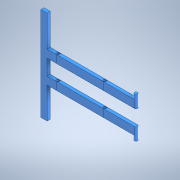
# Autodesk Inventor part: base
Saved by Autodesk Inventor 2022 (Build 260153000, 153)
## iProperties
Created: 2021-12-27
Part Number: base
Material: Stainless Steel
Document SubType Name: Modeling
Designer: G S SHOURIE
Density: 8 g/cm^3
Appearance: Cyan
Mass: 1571.73 g
Surface Area: 614.982 cm^2
Volume: 196.466 cm^3
Author: G S SHOURIE
Autodesk Inventor part; units mm, degrees
ref_plane "YZ Plane" through (0, 0, 0) normal (1, 0, 0) x (0, 1, 0)
ref_plane "XZ Plane" through (0, 0, 0) normal (0, 1, 0) x (-1, 0, 0)
ref_plane "XY Plane" through (0, 0, 0) normal (0, 0, 1) x (1, 0, 0)
sketch "Sketch1" plane through (0, 0, 0) normal (0, 0, 1) x (1, 0, 0)
  line L0 (-150, 150) -> (150, 150)
  line L1 (150, 150) -> (150, -150)
  line L2 (150, -150) -> (-150, -150)
  line L3 (-150, -150) -> (-150, 150)
  point P0 (0, 0)
  dimension "d0" = 300
  dimension "d1" = 300
  dimension "d2" = 150
  dimension "d3" = 150
  constraints: 8 end point, 2 parallel, 1 horizontal, 1 perpendicular
  measures "d0" distance of L0.start L0.end
  measures "d1" distance of L0.end L1.end
  measures "d2" distance from line of L3 point (0, 0)
  measures "d3" distance from line of L0 point (0, 0)
extrude "Extrusion1" add sketch "Sketch1" along normal mid plane 10
sketch "Sketch2" plane through (0, 0, 5) normal (0, 0, 1) x (1, 0, 0)
  line L0 (-130, 25) -> (323.6487, 25)
  line L1 (323.6487, 25) -> (323.6487, -25)
  line L2 (323.6487, -25) -> (-130, -25)
  line L3 (-130, -25) -> (-130, 25)
  point P0 (0, 0)
  dimension "d6" = 50
  dimension "d7" = 25
  dimension "d8" = 130
  constraints: 8 end point, 2 parallel, 1 horizontal, 1 perpendicular
  measures "d6" distance of L0.end L1.end
  measures "d7" distance from line of L0 point (0, 0)
  measures "d8" distance from line of L3 point (0, 0)
extrude "Extrusion2" cut sketch "Sketch2" against normal blind 10
sketch "Sketch3" plane through (0, 0, 5) normal (0, 0, 1) x (1, 0, 0)
  line L0 (170, -50) -> (-130, -50)
  line L1 (-130, -50) -> (-130, -158.2485)
  line L2 (-130, -158.2485) -> (170, -158.2485)
  line L3 (170, -158.2485) -> (170, -50)
  line L4 (150, -25) -> (-130, -25) projected
  point P0 (0, 0)
  dimension "d11" = 300
  dimension "d12" = 130
  dimension "d13" = 25
  constraints: 8 end point, 2 parallel, 1 horizontal, 1 perpendicular
  measures "d11" distance of L1.end L2.end
  measures "d12" distance from line of L1 point (0, 0)
  measures "d13" distance between parallel lines of L0 L4
extrude "Extrusion3" cut sketch "Sketch3" against normal blind 10
mirror "Mirror1" about plane through (0, 0, 0) normal (0, 1, 0) of "Extrusion3"
sketch "Sketch4" plane through (-130, -50, 5) normal (0, -1, 0) x (1, 0, 0)
  point P0 (130, -5)
sketch "Sketch5" plane through (-130, -50, 5) normal (0, -1, 0) x (1, 0, 0)
  point P0 (130, -5)
sketch "Sketch6" plane through (-130, -50, 5) normal (0, -1, 0) x (1, 0, 0)
  point P0 (130, -5)
sketch "Sketch7" plane through (-130, 25, 5) normal (0, -1, 0) x (1, 0, 0)
  circle A0 centre (30, -5) radius 5
  line L0 (0, -10) -> (280, -10) projected
  point P0 (130, -5)
  dimension "d16" = 100
  dimension "d17" = 10
  constraints: 1 centre point, 1 tangent
  measures "d16" distance of A0.centre point (130, -5)
  measures "d17" diameter of A0
extrude "Extrusion4" cut sketch "Sketch7" against normal up to surface (25 mm away)
mirror "Mirror2" about plane through (0, 0, 0) normal (0, 1, 0) of "Extrusion4"
sketch "Sketch8" plane through (-130, -50, 5) normal (0, -1, 0) x (1, 0, 0)
  line L0 (280, 0) -> (280, -10) projected
  circle A0 centre (280, -5) radius 5
  line L1 (0, 0) -> (280, 0) projected
  point P0 (130, -5)
  constraints: 1 centre point, 1 midpoint, 1 tangent
extrude "Extrusion5" add sketch "Sketch8" along normal blind 15
sketch "Sketch9" plane through (-130, -50, 5) normal (0, 1, 0) x (1, 0, 0)
  line L0 (280, 10) -> (280, 0) projected
  circle A0 centre (280, 5) radius 5
  point P0 (130, 5)
  constraints: 1 centre point, 1 midpoint
extrude "Extrusion6" add sketch "Sketch9" along normal up to surface (25 mm away)
mirror "Mirror3" about plane through (0, 0, 0) normal (0, 1, 0) of "Extrusion5", "Extrusion6"
sketch "Sketch10" plane through (-100, 25, 0) normal (0, -1, 0) x (1, 0, 0)
  circle A0 centre (150, 0) radius 5
  line L0 (0, 5) -> (250, 5) projected
  point P0 (100, 0)
  dimension "d24" = 50
  constraints: 1 centre point, 1 tangent
  measures "d24" distance of point (100, 0) A0.centre
extrude "Extrusion7" cut sketch "Sketch10" against normal up to surface (25 mm away)
mirror "Mirror4" about plane through (0, 0, 0) normal (0, 1, 0) of "Extrusion7"
body "Solid1"
